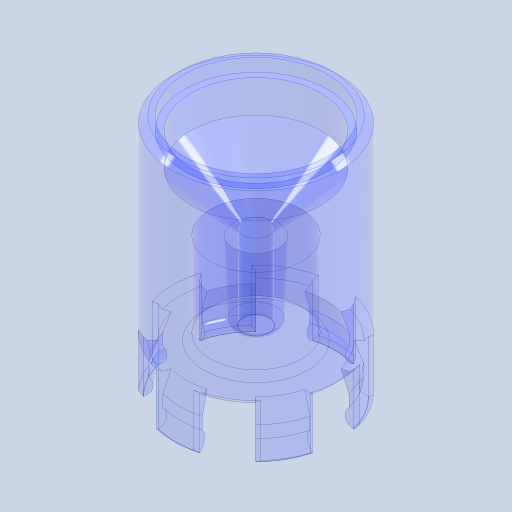
# Autodesk Inventor part: cpd_ultra-TLA100.3_0.7_p4_20230615
Saved by Autodesk Inventor 2024 (Build 280153000, 153)
## iProperties
Created: 2022-02-17
Part Number: cpd_ultra-TLA100.3_0.7_p4_20230615
Material: Generic
Document SubType Name: Modeling
Designer: to172
Density: 1 g/cm^3
Appearance: Clear - Blue
Author: to172
Autodesk Inventor part; units mm, degrees
ref_plane "YZ Plane" through (0, 0, 0) normal (1, 0, 0) x (0, 1, 0)
ref_plane "XZ Plane" through (0, 0, 0) normal (0, 1, 0) x (-1, 0, 0)
ref_plane "XY Plane" through (0, 0, 0) normal (0, 0, 1) x (1, 0, 0)
sketch "Sketch1" plane through (0, 0, 0) normal (0, 0, 1) x (1, 0, 0)
  line L0 (0, 0) -> (0, 12.2836) construction
  line L1 (0, 0) -> (12.7904, 0) construction
  line L2 (3.5, 0) -> (3.5, 7)
  line L3 (3.5, 7) -> (1.725, 7)
  line L4 (1.725, 7) -> (1.725, 1)
  line L5 (1.725, 1) -> (1, 1)
  line L6 (1, 1) -> (1, 7.5)
  line L7 (5, 14) -> (5.5, 14)
  line L8 (5.5, 14) -> (5.5, 15)
  line L9 (5.5, 15) -> (6.4, 15)
  line L10 (6.4, 15) -> (6.4, 0)
  line L11 (6.4, 0) -> (3.5, 0)
  line L12 (1.5155, 1) -> (1.725, 7)
  line L13 (1, 7.5) -> (5, 11.5)
  line L14 (5, 11.5) -> (5, 14)
  dimension "d0" = 15
  dimension "d1" = 6.4
  dimension "d2" = 1.725
  dimension "d3" = 6
  dimension "d4" = 1
  dimension "d5" = 3.5
  dimension "d7" = 1
  dimension "d8" = 7
  dimension "d9" = 6.5
  dimension "d10" = 5.5
  dimension "d28" = 2
  dimension "d30" = 45
  dimension "d31" = 5
  constraints: 30 end point, 8 perpendicular, 3 point on line, 2 vertical, 1 collinear, 1 horizontal, 1 parallel
  measures "d0" distance between parallel lines of L9 L1
  measures "d1" distance between parallel lines of L10 L0
  measures "d2" distance between parallel lines of L4 L0
  measures "d3" distance between parallel lines of L5 L3
  measures "d4" distance between parallel lines of L9 L7
  measures "d5" distance between parallel lines of L2 L0
  measures "d7" distance between parallel lines of L6 L0
  measures "d8" distance between parallel lines of L1 L3
  measures "d9" distance of L5.end L6.end
  measures "d10" distance between parallel lines of L0 L8
  measures "d28" angle of L12 L0
  measures "d30" angle of L0 L13
  measures "d31" distance between parallel lines of L0 L14
revolve "Revolution1" add sketch "Sketch1" angle 360 about axis through (0, 0, 0) along (0, 1, 0) contours L2 L3 L12 L5 L6 L13 L14 L7 L8 L9 L10 L11
sketch "Sketch3" plane through (0, 0, 0) normal (1, 0, 0) x (0, 1, 0)
  line L0 (0, 6.4) -> (0, -6.4) projected
  line L1 (0, -6.4) -> (-3, -6.4)
  line L2 (-3, -5.85) -> (0, -5.85)
  line L3 (0, -5.85) -> (0, -6.4)
  line L4 (-3, -6.4) -> (-3.75, -6.4)
  line L5 (-3.75, -6.4) -> (-3.75, -5.85)
  line L6 (-3.75, -5.85) -> (-3, -5.85)
  line L7 (-4.56, 0) -> (0.76, 0) projected
  circle A0 centre (-3, -6.4) radius 0.8
  line L8 (-1.5, -5.85) -> (0, -5.35)
  line L9 (0, -5.35) -> (0, -5.85)
  point P0 (0, 0)
  point P1 (-2.4191, -5.85)
  point P2 (-3.75, -6.1216)
  dimension "d16" = 0.55
  dimension "d32" = 3.75
  dimension "d33" = 1.6
  dimension "d34" = 0.75
  dimension "d35" = 0.5
  dimension "d36" = 1.5
  constraints: 16 end point, 3 collinear, 2 horizontal, 2 parallel, 2 point on line, 1 centre point, 1 coincident, 1 midpoint, 1 perpendicular
  measures "d16" distance between parallel lines of L2 L1
  measures "d32" distance between parallel lines of L0 L5
  measures "d33" diameter of A0
  measures "d34" distance from line of L5 A0.centre
  measures "d35" distance from line of L8.end L2
  measures "d36" distance from line of L0 L8.start
revolve "Revolution2" add sketch "Sketch3" angle 30 mid plane about axis through (0, -10, 0) along (0, 1, 0) contours L0 L2 L8 | L0 L1 A0 L2 | A0 L1 L4 L5 L6 L2 | L2 L6 A0
chamfer "Chamfer1" distance 0.25 angle 45 3 edges at (-1.6564, -1.875, -6.1819) (1.6564, -1.875, -6.1819) (0, -3.75, -6.4)
pattern_circular "Circular Pattern1" count 6 over 360 about axis through (0, -10, 0) along (0, 1, 0) of "Revolution2", "Chamfer1"
chamfer "Chamfer2" distance 0.5 angle 45 19 edges at (6.1484, 0, -1.7769) (6.3452, 0, -0.8354) (6.3452, 0, 0.8354) (6.1484, 0, 1.7769) (4.613, 0, 4.4362) (3.2, 0, 5.5426) (1.5354, 0, 6.2131) (-4.613, 0, 4.4362) (-3.2, 0, 5.5426) (-1.5354, 0, 6.2131) (-6.1484, 0, -1.7769) (-6.4, 0, 0) (-6.1484, 0, 1.7769) (-3.0911, 0, -5.604) (-4.613, 0, -4.4362) (4.613, 0, -4.4362) (3.0911, 0, -5.604) (-3.5, 0, 0) (-6.4, 15, 0)
fillet "Fillet1" radius 0.5 1 edges at (-1.5155, 1, 0)
body "Solid1"
